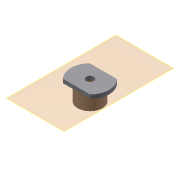
# Autodesk Inventor part: ECoG_holder_cap
Saved by Autodesk Inventor 2014 (Build 180170000, 170)
## iProperties
Created: 2016-07-27
Part Number: ECoG_holder_cap
Material: Generic
Document SubType Name: Modeling
Designer: Camilo
Density: 1 g/cm^3
Appearance: Default
Author: Camilo
Autodesk Inventor part; units mm, degrees
ref_plane "YZ Plane" through (0, 0, 0) normal (1, 0, 0) x (0, 1, 0)
ref_plane "XZ Plane" through (0, 0, 0) normal (0, 1, 0) x (-1, 0, 0)
ref_plane "XY Plane" through (0, 0, 0) normal (0, 0, 1) x (1, 0, 0)
ref_plane "Work Plane1" through (0, 0, 0) normal (0, 0, 1) x (1, 0, 0)
sketch "Sketch1" plane through (0, 0, 0) normal (0, 0, 1) x (1, 0, 0)
  line L0 (2.5, 7.4741) -> (2.5, 6.4741) construction
  arc A0 (2.5, -6.4741) -> (2.5, 6.4741) centre (0, 0) ccw construction
  line L1 (2.5, -6.4741) -> (2.5, -7.4741) construction
  line L2 (2.5, -7.4741) -> (-2.5, -7.4741) construction
  line L3 (-2.5, -7.4741) -> (-2.5, -6.4741) construction
  arc A1 (-2.5, 6.4741) -> (-2.5, -6.4741) centre (0, 0) ccw construction
  line L4 (-2.5, 6.4741) -> (-2.5, 7.4741) construction
  line L5 (-2.5, 7.4741) -> (2.5, 7.4741) construction
  arc A2 (-11, 8.1244) -> (-11, -8.1244) centre (0, 0) ccw construction
  line L6 (-11, -8.1244) -> (-11, -25.94) construction
  line L7 (-11, -25.94) -> (11, -25.94) construction
  line L8 (11, -25.94) -> (11, -8.1244) construction
  arc A3 (11, -8.1244) -> (11, 8.1244) centre (0, 0) ccw construction
  line L9 (11, 25.94) -> (11, 8.1244) construction
  line L10 (-11, 25.94) -> (11, 25.94) construction
  line L11 (-11, 8.1244) -> (-11, 25.94) construction
  line L12 (-7.0828, 6.9741) -> (7.0828, 6.9741)
  line L13 (-7.0828, -6.9741) -> (7.0828, -6.9741)
  arc A4 (-7.0828, 6.9741) -> (-7.0828, -6.9741) centre (0, 0) ccw
  arc A5 (7.0828, -6.9741) -> (7.0828, 6.9741) centre (0, 0) ccw
  point P0 (0, 0)
  dimension "d1" = 0.5
  dimension "d2" = 0.5
  constraints: 4 end point, 4 point on circle, 2 centre point, 2 parallel, 1 coincident
  measures "d1" distance between parallel lines of L5 L12
  measures "d2" distance between parallel lines of L2 L13
extrude "Extrusion1" add sketch "Sketch1" along normal blind 2
sketch "Sketch2" plane through (0, 0, 0) normal (0, 0, -1) x (-1, 0, 0)
  line L0 (-2.5, 7.4741) -> (-2.5, 6.4741) construction
  arc A0 (-2.5, 6.4741) -> (-2.5, -6.4741) centre (0, 0) ccw construction
  line L1 (-2.5, -6.4741) -> (-2.5, -7.4741) construction
  line L2 (-2.5, -7.4741) -> (2.5, -7.4741) construction
  line L3 (2.5, -7.4741) -> (2.5, -6.4741) construction
  arc A1 (2.5, -6.4741) -> (2.5, 6.4741) centre (0, 0) ccw construction
  line L4 (2.5, 6.4741) -> (2.5, 7.4741) construction
  line L5 (2.5, 7.4741) -> (-2.5, 7.4741) construction
  arc A2 (11, -8.1244) -> (11, 8.1244) centre (0, 0) ccw construction
  line L6 (11, -8.1244) -> (11, -25.94) construction
  line L7 (11, -25.94) -> (-11, -25.94) construction
  line L8 (-11, -25.94) -> (-11, -8.1244) construction
  arc A3 (-11, 8.1244) -> (-11, -8.1244) centre (0, 0) ccw construction
  line L9 (-11, 25.94) -> (-11, 8.1244) construction
  line L10 (11, 25.94) -> (-11, 25.94) construction
  line L11 (11, 8.1244) -> (11, 25.94) construction
  circle A4 centre (0, 0) radius 6.44
  circle A5 centre (0, 0) radius 4.44
  dimension "d5" = 0.5
  dimension "d6" = 2
  constraints: 2 centre point, 2 coincident
  measures "d5" radial gap between concentric circles of A1 A4
  measures "d6" radial gap between concentric circles of A4 A5
extrude "Extrusion2" add sketch "Sketch2" along normal blind 8
sketch "Sketch3" plane through (0, 0, 2) normal (0, 0, 1) x (1, 0, 0)
  arc A0 (7.0828, -6.9741) -> (7.0828, 6.9741) centre (0, 0) ccw projected
  circle A1 centre (0, 0) radius 2
  constraints: 1 centre point, 1 coincident
extrude "Extrusion3" cut sketch "Sketch3" against normal through all
body "Solid1"
